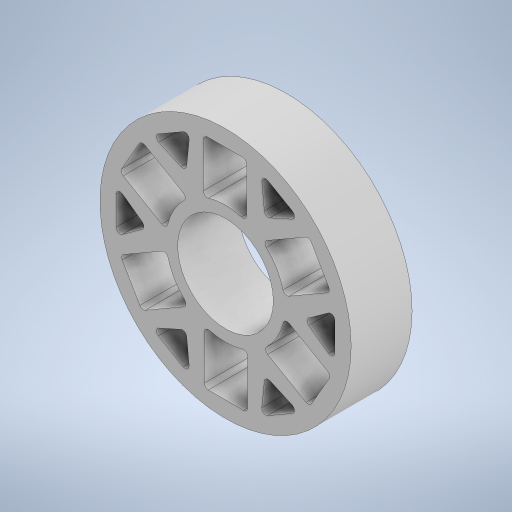
# Autodesk Inventor part: EXPANDED FLEX WHEEL
Saved by Autodesk Inventor 2024 (Build 280153000, 153)
## iProperties
Created: 2023-09-29
Part Number: EXPANDED FLEX WHEEL
Material: Generic
Document SubType Name: Modeling
Designer: Robodox
Density: 1 g/cm^3
Appearance: Default
Author: Robodox
Autodesk Inventor part; units mm, degrees
ref_plane "YZ Plane" through (0, 0, 0) normal (1, 0, 0) x (0, 1, 0)
ref_plane "XZ Plane" through (0, 0, 0) normal (0, 1, 0) x (-1, 0, 0)
ref_plane "XY Plane" through (0, 0, 0) normal (0, 0, 1) x (1, 0, 0)
sketch "Sketch1" plane through (0, 0, 0) normal (0, 0, 1) x (1, 0, 0)
  circle A0 centre (0, 0) radius 19.939
  circle A1 centre (0, 0) radius 52.3875
  line L0 (-9.2075, 22.9897) -> (-9.2075, 45.5957)
  line L1 (-9.2075, 45.5957) -> (8.8265, 45.5957)
  line L2 (8.8265, 45.5957) -> (8.8265, 23.1387)
  line L3 (-44.0908, 14.8239) -> (-35.0738, 30.4418)
  line L4 (-35.0738, 30.4418) -> (-15.6254, 19.2133)
  line L5 (-24.5134, 3.5209) -> (-44.0908, 14.8239)
  line L6 (-34.8833, -30.7718) -> (-43.9003, -15.1539)
  line L7 (-43.9003, -15.1539) -> (-24.4519, -3.9254)
  line L8 (-15.3059, -19.4688) -> (-34.8833, -30.7718)
  line L9 (9.2075, -45.5957) -> (-8.8265, -45.5957)
  line L10 (-8.8265, -45.5957) -> (-8.8265, -23.1387)
  line L11 (9.2075, -22.9897) -> (9.2075, -45.5957)
  line L12 (44.0908, -14.8239) -> (35.0738, -30.4418)
  line L13 (35.0738, -30.4418) -> (15.6254, -19.2133)
  line L14 (24.5134, -3.5209) -> (44.0908, -14.8239)
  line L15 (34.8833, 30.7718) -> (43.9003, 15.1539)
  line L16 (43.9003, 15.1539) -> (24.4519, 3.9254)
  line L17 (15.3059, 19.4688) -> (34.8833, 30.7718)
  arc A2 (8.8265, 23.1387) -> (-9.2075, 22.9897) centre (0, 0) ccw
  arc A3 (-15.6254, 19.2133) -> (-24.5134, 3.5209) centre (0, 0) ccw
  arc A4 (24.4519, 3.9254) -> (15.3059, 19.4688) centre (0, 0) ccw
  arc A5 (15.6254, -19.2133) -> (24.5134, -3.5209) centre (0, 0) ccw
  arc A6 (-24.4519, -3.9254) -> (-15.3059, -19.4688) centre (0, 0) ccw
  arc A7 (-8.8265, -23.1387) -> (9.2075, -22.9897) centre (0, 0) ccw
  line L18 (-45.5802, 9.2075) -> (-32.8802, 0)
  line L19 (-32.8802, 0) -> (-45.5802, -9.2075)
  line L20 (-45.5802, -9.2075) -> (-45.5802, 9.2075)
  line L21 (-30.764, -34.8699) -> (-16.4401, -28.4751)
  line L22 (-14.8162, -44.0774) -> (-30.764, -34.8699)
  line L23 (-16.4401, -28.4751) -> (-14.8162, -44.0774)
  line L24 (14.8162, -44.0774) -> (16.4401, -28.4751)
  line L25 (30.764, -34.8699) -> (14.8162, -44.0774)
  line L26 (16.4401, -28.4751) -> (30.764, -34.8699)
  line L27 (45.5802, -9.2075) -> (32.8802, 0)
  line L28 (45.5802, 9.2075) -> (45.5802, -9.2075)
  line L29 (32.8802, 0) -> (45.5802, 9.2075)
  line L30 (30.764, 34.8699) -> (16.4401, 28.4751)
  line L31 (14.8162, 44.0774) -> (30.764, 34.8699)
  line L32 (16.4401, 28.4751) -> (14.8162, 44.0774)
  line L33 (-14.8162, 44.0774) -> (-16.4401, 28.4751)
  line L34 (-30.764, 34.8699) -> (-14.8162, 44.0774)
  line L35 (-16.4401, 28.4751) -> (-30.764, 34.8699)
  dimension "d0" = 39.878
  dimension "d3" = 104.775
  dimension "d38" = 22.606
  dimension "d39" = 18.034
  dimension "d40" = 9.2075
  dimension "d41" = 360
  dimension "d42" = 9.2075
  dimension "d43" = 9.2075
  dimension "d44" = 9.2075
  dimension "d45" = 12.7
  dimension "d46" = 12.7
  dimension "d49" = 360
  constraints: 72 end point, 12 point on circle, 8 centre point, 4 coincident, 2 perpendicular, 1 vertical, 80 other
  measures "d0" diameter of A0
  measures "d3" diameter of A1
  measures "d38" distance of L0.start L0.end
  measures "d39" distance of L0.end L1.end
  measures "d40" distance from line of point (0, 0) L0
  measures "d42" vertical distance of point (0, 0) L18.start
  measures "d43" vertical distance of point (0, 0) L19.end
  measures "d44" vertical distance of L18.start L18.end
  measures "d45" horizontal distance of L18.end L19.end
  measures "d46" horizontal distance of L18.start L18.end
extrude "Extrusion2" add sketch "Sketch1" along normal blind 25.4
fillet "Fillet1" radius 1.651 42 edges at (-15.6254, 19.2133, 12.7) (8.8265, 45.5957, 12.7) (30.764, 34.8699, 12.7) (43.9003, 15.1539, 12.7) (-32.8802, 0, 12.7) (-15.3059, -19.4688, 12.7) (-44.0908, 14.8239, 12.7) (-30.764, 34.8699, 12.7) (15.3059, 19.4688, 12.7) (15.6254, -19.2133, 12.7) (32.8802, 0, 12.7) (-30.764, -34.8699, 12.7) (-43.9003, -15.1539, 12.7) (-9.2075, 22.9897, 12.7) (16.4401, 28.4751, 12.7) (24.4519, 3.9254, 12.7) (9.2075, -45.5957, 12.7) (35.0738, -30.4418, 12.7) (45.5802, -9.2075, 12.7) (-14.8162, -44.0774, 12.7) (-24.5134, 3.5209, 12.7) (8.8265, 23.1387, 12.7) (-16.4401, 28.4751, 12.7) (-34.8833, -30.7718, 12.7) (-8.8265, -45.5957, 12.7) (14.8162, -44.0774, 12.7) (-45.5802, -9.2075, 12.7) (-45.5802, 9.2075, 12.7) (-35.0738, 30.4418, 12.7) (-9.2075, 45.5957, 12.7) (-8.8265, -23.1387, 12.7) (24.5134, -3.5209, 12.7) (16.4401, -28.4751, 12.7) (14.8162, 44.0774, 12.7) (9.2075, -22.9897, 12.7) (44.0908, -14.8239, 12.7) (30.764, -34.8699, 12.7) (34.8833, 30.7718, 12.7) (45.5802, 9.2075, 12.7) (-16.4401, -28.4751, 12.7) (-24.4519, -3.9254, 12.7) (-14.8162, 44.0774, 12.7)
body "Solid2"
